Autodesk Fusion 360 part; units mm, degrees
(part 2 of 2)
sketch "Sketch2 (5)" plane through (0, -14.283858, -47.665117) normal (0, -0.287059, -0.957913) x (1, 0, 0) in component "Stone Harbor Pipe Holder 7\""
  circle A0 centre (5.32, 118.742647) radius 1.7
  line L0 (7.043146, -11.757353) -> (7.043146, 151.104016)
  line L1 (7.043146, 151.104016) -> (3.956854, 151.104016)
  line L2 (3.956854, 151.104016) -> (3.956854, -11.757353)
  line L3 (3.956854, -11.757353) -> (7.043146, -11.757353)
  line L4 (5.5, 151.104016) -> (5.5, -11.757353) construction
  circle A1 centre (5.5, 52.242647) radius 1.7
  dimension "d211_1" = 3.4
  dimension "d239" = 3.4
  dimension "d240" = 64
  dimension "d241" = 130.5
  measures "d211_1" diameter of A0
  measures "d239" diameter of A1
extrude "Extrude2'''''''" cut sketch "Sketch2 (5)" against normal blind 10 contours A0 L2 | A0 L2 | L0 L2 A1 | L2 A1 | L0 A1 picked at (6.238318, 118.25061) picked at (3.913423, 118.47192) picked at (5.936592, 52.004903) picked at (3.92801, 52.403944) picked at (7.07199, 52.403944) bodies 17 in component "Stone Harbor Pipe Holder 7\""
sketch "Sketch1 (14)" plane through (0, 0, 0) normal (1, 0, 0) x (0, 1, 0) in component "Knape Vogt Pipe Holder 7\""
  line L0 (-173.859658, 11.32859) -> (-173.859658, -2.47141) construction
  line L1 (-17.859658, 9.32859) -> (-17.859658, -4.47141) construction
  circle A0 centre (-173.859658, 11.32859) radius 10.05
  circle A1 centre (-17.859658, 9.32859) radius 10.05
  line L2 (-31.659658, -3.47141) -> (-31.659658, 9.32859)
  circle A2 centre (-173.859658, 11.32859) radius 13.8
  line L3 (-4.059658, -47.67141) -> (-4.059658, 9.32859)
  circle A3 centre (-17.859658, 9.32859) radius 13.8
  line L4 (-160.059658, 11.32859) -> (-102.238094, -3.47141)
  line L5 (-173.859658, 11.32859) -> (-160.059658, 11.32859) construction
  line L6 (-161.207894, -7.447768) -> (-164.080996, -2.47141)
  line L7 (-164.080996, -2.47141) -> (-173.859658, -2.47141)
  line L8 (-31.659658, -3.47141) -> (-102.238094, -3.47141)
  line L9 (-4.059658, -47.67141) -> (-161.207894, -7.447768)
  line L10 (-9.021337, -14.67141) -> (-9.021337, -24.67141)
  line L11 (-9.021337, -24.67141) -> (-4.059658, -28.834753)
  line L12 (-4.059658, -10.508067) -> (-9.021337, -14.67141)
  point P0 (-9.021337, -19.67141)
  dimension "d168_1_1" = 20.1
  dimension "d169_1_1" = 27.6
  dimension "d170_1_1" = 20.1
  dimension "d171_1_1" = 27.6
  dimension "d216_1" = 57
  dimension "d217_1" = 12.8
  dimension "d233_1" = 120
  dimension "d234_1" = 9.778663
  dimension "d235_1" = 5.746204
  dimension "d237_1" = 1
  dimension "d243" = 156
  dimension "d251" = 130
  dimension "d252" = 10
  dimension "d253" = 29
  constraint concentric A1 A3
  constraint concentric A0 A2
  constraint vertical L1
  constraint tangent L3 A3
  constraint vertical L3
  constraint vertical L2
  constraint tangent L2 A3
  constraint vertical L0
  constraint horizontal L5
  constraint tangent A2 L7
  constraint perpendicular L2 L8
  constraint horizontal L7
  constraint parallel L4 L9
  constraint equal L11 L12
  constraint vertical L10
  measures "d168_1_1" diameter of A1
  measures "d169_1_1" diameter of A3
  measures "d170_1_1" diameter of A0
  measures "d171_1_1" diameter of A2
  measures "d233_1" angle of L6 L7
  measures "d237_1" distance of L7 L8
  measures "d251" angle of L10 L12
extrude "Extrude1'''''''''''''" add sketch "Sketch1 (14)" along normal blind 8.8 separate body contours L2 A2 L3 A3 L4 L6 L7 L8 L9 L10 L11 L12 | A3 | A2 picked at (-45.985803, -18.204743) picked at (-5.361037, 8.642996) picked at (-174.784964, -1.162254) makes body 18 in component "Knape Vogt Pipe Holder 7\""
move_face "OffsetFaces1'''" offset -0.3 1 faces at (0, -45.985803, -18.204743) on bodies 18 in component "Knape Vogt Pipe Holder 7\""
move_face "OffsetFaces2'''" offset -0.3 1 faces at (8.8, -45.985803, -18.204743) on bodies 18 in component "Knape Vogt Pipe Holder 7\""
fillet "Fillet1'''''" radius 8 1 edges at (4.4, -31.659658, -3.47141) on bodies 18 in component "Knape Vogt Pipe Holder 7\""
fillet "Fillet2'''''" radius 100 1 edges at (4.4, -102.238094, -3.47141) on bodies 18 in component "Knape Vogt Pipe Holder 7\""
fillet "Fillet3'''''" radius 10 1 edges at (4.4, -160.059658, 11.32859) on bodies 18 in component "Knape Vogt Pipe Holder 7\""
fillet "Fillet4'''''" radius 3 2 edges at (4.4, -164.080996, -2.47141) (4.4, -161.207894, -7.447768) on bodies 18 in component "Knape Vogt Pipe Holder 7\""
chamfer "Chamfer1'''" distance 2 angle 45 30 edges at (0.3, -162.527033, -5.162952) (0.3, -161.053923, -7.244762) (0.3, -82.022288, -27.716105) (0.3, -4.059658, -0.589738) (0.3, -4.059658, -38.253081) (0.3, -17.859658, 23.12859) (0.3, -31.659658, 6.92859) (0.3, -34.002804, -1.128264) (0.3, -64.651389, -3.47141) (0.3, -102.139367, -2.687556) (0.3, -134.205184, 4.710883) (0.3, -158.207246, 12.048824) (0.3, -185.162022, 19.246707) (0.3, -169.836352, -2.47141) (0.3, -164.313046, -2.873333) (8.5, -162.527033, -5.162952) (8.5, -164.313046, -2.873333) (8.5, -169.836352, -2.47141) (8.5, -185.162022, 19.246707) (8.5, -158.207246, 12.048824) (8.5, -134.205184, 4.710883) (8.5, -102.139367, -2.687556) (8.5, -64.651389, -3.47141) (8.5, -34.002804, -1.128264) (8.5, -31.659658, 6.92859) (8.5, -17.859658, 23.12859) (8.5, -4.059658, -38.253081) (8.5, -4.059658, -0.589738) (8.5, -82.022288, -27.716105) (8.5, -161.053923, -7.244762) on bodies 18 in component "Knape Vogt Pipe Holder 7\""
fillet "Fillet5''''" radius 4 30 edges at (2.3, -162.527033, -5.162952) (2.3, -164.313046, -2.873333) (2.3, -169.836352, -2.47141) (2.3, -185.162022, 19.246707) (2.3, -158.207246, 12.048824) (2.3, -134.205184, 4.710883) (2.3, -102.139367, -2.687556) (2.3, -64.651389, -3.47141) (2.3, -34.002804, -1.128264) (2.3, -31.659658, 6.92859) (2.3, -17.859658, 23.12859) (2.3, -4.059658, -0.589738) (2.3, -4.059658, -38.253081) (2.3, -161.053923, -7.244762) (2.3, -82.022288, -27.716105) (6.5, -4.059658, -38.253081) (6.5, -4.059658, -0.589738) (6.5, -17.859658, 23.12859) (6.5, -31.659658, 6.92859) (6.5, -34.002804, -1.128264) (6.5, -64.651389, -3.47141) (6.5, -102.139367, -2.687556) (6.5, -134.205184, 4.710883) (6.5, -158.207246, 12.048824) (6.5, -185.162022, 19.246707) (6.5, -169.836352, -2.47141) (6.5, -164.313046, -2.873333) (6.5, -162.527033, -5.162952) (6.5, -161.053923, -7.244762) (6.5, -82.022288, -27.716105) on bodies 18 in component "Knape Vogt Pipe Holder 7\""
sketch "Sketch2 (6)" plane through (0, -11.701321, -45.715451) normal (0, -0.247966, -0.968769) x (1, 0, 0) in component "Knape Vogt Pipe Holder 7\""
  circle A0 centre (5.32, 140.111985) radius 1.7
  line L0 (4.843146, -7.888015) -> (4.843146, 153.063975)
  line L1 (4.843146, 153.063975) -> (3.956854, 153.063975)
  line L2 (3.956854, 153.063975) -> (3.956854, -7.888015)
  line L3 (3.956854, -7.888015) -> (4.843146, -7.888015)
  line L4 (4.4, 153.063975) -> (4.4, -7.888015) construction
  circle A1 centre (4.4, 38.111985) radius 1.7
  dimension "d211_1_1" = 3.4
  dimension "d239_1" = 3.4
  dimension "d240_1" = 46
  dimension "d241_1" = 148
  measures "d211_1_1" diameter of A0
  measures "d239_1" diameter of A1
extrude "Extrude2''''''''" cut sketch "Sketch2 (6)" against normal blind 10 contours A0 L0 | A0 L0 L2 | A0 L2 | L0 A1 | L0 L2 A1 | L2 A1 picked at (5.563004, 140.192575) picked at (4.70942, 140.597219) picked at (3.913423, 140.382713) picked at (5.682624, 38.088405) picked at (4.547715, 38.65906) picked at (3.513224, 37.899967) bodies 18 in component "Knape Vogt Pipe Holder 7\""
move_body "Move1" bodies 18 to x (1, 0, 0) y (0, 1, 0) z (0, 0, 1) at (0, 0, -130) in component "Knape Vogt Pipe Holder 7\""
component "GROUND Spool Bambu Lab 1kg" placed x (1, 0, 0) y (0, 1, 0) z (0, 0, 1) at (0, 0, 0)
component "Spool Bambu Lab 1kg (1)" placed x (1, 0, 0) y (0, 1, 0) z (0, 0, 1) at (15, -93.76622, 228.302243)
component "Box Bambu Lab Refill" placed x (1, 0, 0) y (0, 0.9998477, -0.01745241) z (0, 0.01745241, 0.9998477) at (115, -87.045072, 258.435301)
component "Box Bambu Lab with Spool" placed x (1, 0, 0) y (0, 0.9998477, -0.01745241) z (0, 0.01745241, 0.9998477) at (215, -96.94756, 264.108987)
component "Box Polymaker" placed x (1, 0, 0) y (0, 0.9998477, -0.01745241) z (0, 0.01745241, 0.9998477) at (315, -98.438606, 264.63509)
component "Shelf Vertical Track 48\"" placed x (1, 0, 0) y (0, 1, 0) z (0, 0, 1) at (0, 0, 0)
component "Shelf Bracket 9.53\"" placed x (1, 0, 0) y (0, 1, 0) z (0, 0, 1) at (-5.09, 11.1, -563.066528)
component "Lowes Shelf Bracket 9.53\" (1)" placed x (1, 0, 0) y (0, 1, 0) z (0, 0, 1) at (-5.32, 11.1, 135.931444)
component "Pipe Holder" placed x (1, 0, 0) y (0, 1, 0) z (0, 0, 1) at (-5.09, 11.1, 136.933)
component "Lowes Pipe Holder 6.75\"" placed x (1, 0, 0) y (0, 1, 0) z (0, 0, 1) at (-4.79, 11.1, 135.873027)
component "Pipe" placed x (1, 0, 0) y (0, 1, 0) z (0, 0, 1) at (-196.26, -19.6, 150.633)
component "Pipe" placed x (1, 0, 0) y (0, 1, 0) z (0, 0, 1) at (-196.26, -216.913428, 152.633)
component "Pipe" placed x (1, 0, 0) y (0, 1, 0) z (0, 0, 1) at (-196.26, -172.7, 150.702)
component "Pipe" placed x (1, 0, 0) y (0, 1, 0) z (0, 0, 1) at (-196.26, -16.7, 148.702)
component "Shelf Board 10\" Depth" placed x (1, 0, 0) y (0, 1, 0) z (0, 0, 1) at (-196.26, 0, -213.729528)
component "Shelf Board 10\" Depth" placed x (1, 0, 0) y (0, 1, 0) z (0, 0, 1) at (-196.26, 0, -563.066528)
component "Shelf Bracket 9.53\"" placed x (1, 0, 0) y (0, 1, 0) z (0, 0, 1) at (-5.09, 11.1, -213.729528)
component "Shelf Bracket 9.53\"" placed x (1, 0, 0) y (0, 1, 0) z (0, 0, 1) at (-5.09, 11.1, 136.933472)
component "Shelf Vertical Track 48\"" placed x (1, 0, 0) y (0, 1, 0) z (0, 0, 1) at (406.4, 0, 0)
component "Shelf Vertical Track 48\"" placed x (1, 0, 0) y (0, 1, 0) z (0, 0, 1) at (812.8, 0, 0)
component "Shelf Vertical Track 48\"" placed x (1, 0, 0) y (0, 1, 0) z (0, 0, 1) at (1219.2, 0, 0)
component "Shelf Vertical Track 48\"" placed x (1, 0, 0) y (0, 1, 0) z (0, 0, 1) at (1625.6, 0, 0)
component "Shelf Vertical Track 48\"" placed x (1, 0, 0) y (0, 1, 0) z (0, 0, 1) at (2032, 0, 0)
component "Shelf Bracket 9.53\"" placed x (1, 0, 0) y (0, 1, 0) z (0, 0, 1) at (401.31, 11.1, -563.066528)
component "Shelf Bracket 9.53\"" placed x (1, 0, 0) y (0, 1, 0) z (0, 0, 1) at (401.31, 11.1, -213.729528)
component "Shelf Bracket 9.53\"" placed x (1, 0, 0) y (0, 1, 0) z (0, 0, 1) at (807.71, 11.1, -563.066528)
component "Shelf Bracket 9.53\"" placed x (1, 0, 0) y (0, 1, 0) z (0, 0, 1) at (807.71, 11.1, -213.729528)
component "Shelf Bracket 9.53\"" placed x (1, 0, 0) y (0, 1, 0) z (0, 0, 1) at (1214.11, 11.1, -563.066528)
component "Shelf Bracket 9.53\"" placed x (1, 0, 0) y (0, 1, 0) z (0, 0, 1) at (1214.11, 11.1, -213.729528)
component "Shelf Bracket 9.53\"" placed x (1, 0, 0) y (0, 1, 0) z (0, 0, 1) at (1620.51, 11.1, -563.066528)
component "Shelf Bracket 9.53\"" placed x (1, 0, 0) y (0, 1, 0) z (0, 0, 1) at (1620.51, 11.1, -213.729528)
component "Shelf Bracket 9.53\"" placed x (1, 0, 0) y (0, 1, 0) z (0, 0, 1) at (2026.91, 11.1, -563.066528)
component "Shelf Bracket 9.53\"" placed x (1, 0, 0) y (0, 1, 0) z (0, 0, 1) at (2026.91, 11.1, -213.729528)
component "Lowes Shelf Bracket 9.53\" (1)" placed x (1, 0, 0) y (0, 1, 0) z (0, 0, 1) at (401.08, 11.1, 135.931444)
component "Lowes Pipe Holder 6.75\"" placed x (1, 0, 0) y (0, 1, 0) z (0, 0, 1) at (401.61, 11.1, 135.873027)
component "Lowes Shelf Bracket 9.53\" (1)" placed x (1, 0, 0) y (0, 1, 0) z (0, 0, 1) at (807.48, 11.1, 135.931444)
component "Lowes Pipe Holder 6.75\"" placed x (1, 0, 0) y (0, 1, 0) z (0, 0, 1) at (808.01, 11.1, 135.873027)
component "Lowes Shelf Bracket 9.53\" (1)" placed x (1, 0, 0) y (0, 1, 0) z (0, 0, 1) at (1213.88, 11.1, 135.931444)
component "Lowes Pipe Holder 6.75\"" placed x (1, 0, 0) y (0, 1, 0) z (0, 0, 1) at (1214.41, 11.1, 135.873027)
component "Lowes Shelf Bracket 9.53\" (1)" placed x (1, 0, 0) y (0, 1, 0) z (0, 0, 1) at (1620.28, 11.1, 135.931444)
component "Lowes Pipe Holder 6.75\"" placed x (1, 0, 0) y (0, 1, 0) z (0, 0, 1) at (1620.81, 11.1, 135.873027)
component "Lowes Shelf Bracket 9.53\" (1)" placed x (1, 0, 0) y (0, 1, 0) z (0, 0, 1) at (2026.68, 11.1, 135.931444)
component "Lowes Pipe Holder 6.75\"" placed x (1, 0, 0) y (0, 1, 0) z (0, 0, 1) at (2027.21, 11.1, 135.873027)
component "Stone Harbor Pipe Holder 7\"" placed x (1, 0, 0) y (0, 1, 0) z (0, 0, 1) at (0, 0, 0)
component "Knape Vogt Pipe Holder 7\"" placed x (1, 0, 0) y (0, 1, 0) z (0, 0, 1) at (0, 0, 0)
equation "d30 = 915 mm + 333 mm"
equation "d31 = track_metal_thickness"
equation "d32 = track_metal_thickness"
equation "track_metal_thickness = 1.9 mm"
equation "d36 = 7.2 mm + 0.5 mm"
equation "d49 = -track_metal_thickness"
equation "d51 = 16.9 mm - track_metal_thickness"
equation "d63 = 16\""
equation "d80 = -track_metal_thickness"
equation "d82 = track_metal_thickness"
equation "d83 = 13.74 mm - 2 * track_metal_thickness"
equation "d86 = track_metal_thickness"
equation "d88 = track_metal_thickness"
equation "rod_outer_diameter = 19.6 mm"
equation "rod_inner_diameter = 17.3 mm"
equation "d116 = rod_outer_diameter"
equation "d117 = rod_outer_diameter + 8 mm"
equation "d118 = rod_outer_diameter"
equation "d119 = rod_outer_diameter + 8 mm"
equation "m4_screw_hole_diam = 3.4 mm"
equation "d142 = m4_screw_hole_diam"
equation "d143 = m4_screw_hole_diam"
equation "m4_screw_hole_depth = 10 mm"
equation "d145 = -m4_screw_hole_depth"
equation "d147 = rod_outer_diameter - 0.3 mm"
equation "d148 = rod_inner_diameter"
equation "d149 = 90\""
equation "d158 = 72\""
equation "d80_1 = -bracket_metal_thickness"
equation "d82_1 = bracket_metal_thickness"
equation "d83_1 = 13 mm - 2 * bracket_metal_thickness"
equation "d86_1 = bracket_metal_thickness"
equation "d88_1 = bracket_metal_thickness"
equation "d168 = holder_hole_diameter"
equation "d169 = rod_outer_diameter + 8 mm"
equation "d170 = holder_hole_diameter"
equation "d171 = rod_outer_diameter + 8 mm"
equation "bracket_metal_thickness = 1.18 mm"
equation "d210 = m4_screw_hole_diam"
equation "d211 = m4_screw_hole_diam"
equation "d212 = -m4_screw_hole_depth"
equation "holder_hole_diameter = rod_outer_diameter + 0.5 mm"
equation "d168_1 = holder_hole_diameter"
equation "d169_1 = rod_outer_diameter + 8 mm"
equation "d170_1 = holder_hole_diameter"
equation "d171_1 = rod_outer_diameter + 8 mm"
equation "d211_1 = m4_screw_hole_diam"
equation "d212_1 = -m4_screw_hole_depth"
equation "d239 = m4_screw_hole_diam"
equation "d168_1_1 = holder_hole_diameter"
equation "d169_1_1 = rod_outer_diameter + 8 mm"
equation "d170_1_1 = holder_hole_diameter"
equation "d171_1_1 = rod_outer_diameter + 8 mm"
equation "d211_1_1 = m4_screw_hole_diam"
equation "d212_1_1 = -m4_screw_hole_depth"
equation "d239_1 = m4_screw_hole_diam"
named bodies: "Frame", "Spool Core"
